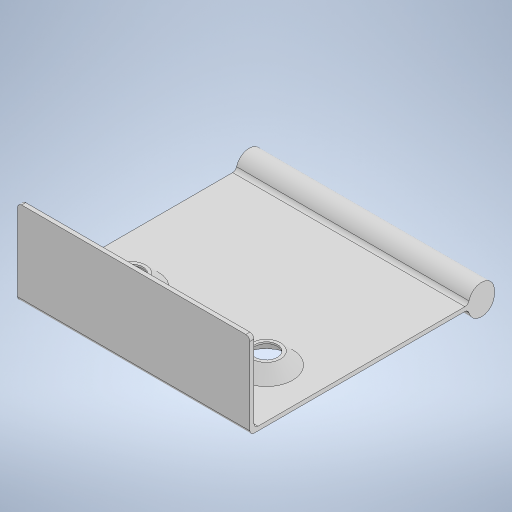
# Autodesk Inventor part: Handle V1
Saved by Autodesk Inventor 2023.4 (Build 274418000, 418)
## iProperties
Created: 2024-05-16
Part Number: Handle V1
Material: Generic
Document SubType Name: Modeling
Designer: Nathan Cai
Density: 1 g/cm^3
Appearance: Default
Author: Nathan Cai
Autodesk Inventor part; units mm, degrees
ref_plane "YZ Plane" through (0, 0, 0) normal (1, 0, 0) x (0, 1, 0)
ref_plane "XZ Plane" through (0, 0, 0) normal (0, 1, 0) x (-1, 0, 0)
ref_plane "XY Plane" through (0, 0, 0) normal (0, 0, 1) x (1, 0, 0)
sketch "Sketch1" plane through (0, 0, 0) normal (0, 1, 0) x (-1, 0, 0)
  line L0 (28.5, 30) -> (-28.5, 30)
  line L1 (-28.5, 30) -> (-28.5, -30)
  line L2 (-28.5, -30) -> (28.5, -30)
  line L3 (28.5, -30) -> (28.5, 30)
  line L4 (28.5, 30) -> (-28.5, -30) construction
  line L5 (-28.5, 30) -> (28.5, -30) construction
  point P0 (0, 0)
  dimension "d0" = 57
  dimension "d1" = 60
  constraints: 12 end point, 2 midpoint, 2 parallel, 1 horizontal, 1 perpendicular
  measures "d0" distance of L2.end L1.end
  measures "d1" distance of L1.end L0.end
extrude "Extrusion1" add sketch "Sketch1" along normal blind 1
sketch "Sketch2" plane through (0, 1, 0) normal (0, 1, 0) x (1, 0, 0)
  line L0 (-28.5, 30) -> (-28.5, -30) projected
  line L1 (28.5, -30) -> (28.5, 30) projected
  line L2 (-28.5, -30) -> (28.5, -30)
  line L3 (28.5, -30) -> (28.5, -29)
  line L4 (28.5, -29) -> (-28.5, -29)
  line L5 (-28.5, -29) -> (-28.5, -30)
  point P0 (0, 0)
  dimension "d4" = 1
  constraints: 8 end point, 2 parallel, 1 horizontal, 1 perpendicular, 1 point on line
  measures "d4" distance of L3.end L2.end
extrude "Extrusion2" add sketch "Sketch2" along normal blind 20
sketch "Sketch3" plane through (0, 1, 0) normal (0, 1, 0) x (1, 0, 0)
  line L0 (-28.5, 30) -> (-28.5, -30) projected
  line L1 (-28.5, -14) -> (28.5, -14) construction
  line L2 (28.5, -30) -> (28.5, 30) projected
  line L3 (28.5, -29) -> (-28.5, -29) projected
  line L4 (0, -29) -> (0, 22.5) construction
  circle A0 centre (-16.5, -14) radius 6.5
  circle A1 centre (16.5, -14) radius 6.5
  point P0 (0, 0)
  dimension "d7" = 15
  dimension "d8" = 13
  dimension "d9" = 12
  constraints: 4 end point, 3 point on line, 2 centre point, 1 horizontal, 1 midpoint, 1 symmetric about line, 1 vertical, 1 other
  measures "d7" distance between parallel lines of L3 L1
  measures "d8" diameter of A0
  measures "d9" distance from line of L0 A0.centre
extrude "Extrusion3" add sketch "Sketch3" along normal blind 3 draft -45
sketch "Sketch4" plane through (0, 0, 0) normal (0, -1, 0) x (1, 0, 0)
  circle A0 centre (16.5, 14) radius 3.5 projected
  circle A1 centre (-16.5, 14) radius 3.5 projected
  circle A2 centre (16.5, 14) radius 3.5 projected
  circle A3 centre (-16.5, 14) radius 3.5 projected
  point P0 (0, 0)
  constraints: 2 coincident
hole "Hole1" at (16.5, 0, 14) at (-16.5, 0, 14) direction (0, 1, 0) diameter 5.5118 end through all countersink diameter 12.7 countersink angle 90 clearance for "Flat Head Machine Screw" size "M5" standard "Ansi Metric M Profile"
fillet "Fillet1" radius 1 2 edges at (0, 1, 29) (0, 0, 30)
sketch "Sketch5" plane through (28.5, 0, 29) normal (1, 0, 0) x (0, 0, -1)
  line L0 (59, 1) -> (1, 1) projected
  arc A0 (59, 1) -> (52.65, 1) centre (55.825, 1) ccw
  line L1 (59, 0) -> (0, 0) projected
  arc A1 (52.65, 0) -> (59, 0) centre (55.825, 0) ccw
  point P0 (29, 0)
  dimension "d20" = 6.35
  dimension "d24" = 6.35
  constraints: 5 point on circle, 5 point on line, 2 centre point, 1 end point
  measures "d20" diameter of A0
  measures "d24" diameter of A1
extrude "Extrusion4" add sketch "Sketch5" against normal up to surface (57 mm away)
fillet "Fillet2" radius 1 5 edges at (0, 1, -23.65) (0, 0, -30) (28.5, 21, 29.5) (-28.5, 21, 29.5) (0, 0, -23.65)
equation "\"d24\" = d20"
body "Solid1"
